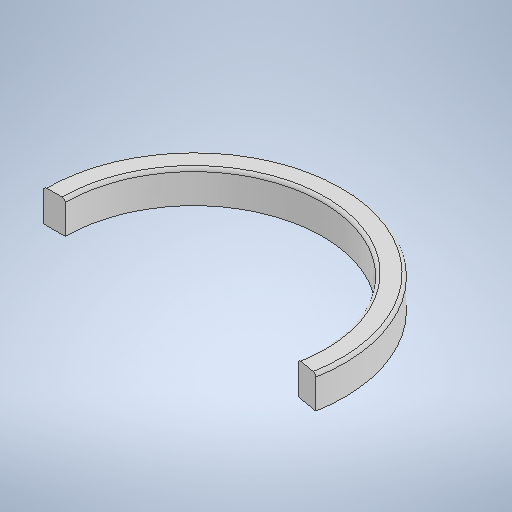
# Autodesk Inventor part: InertiaKitInner
Saved by Autodesk Inventor 2025 (Build 290162000, 162)
## iProperties
Created: 2026-01-08
Part Number: InertiaKitInner
Material: Generic
Document SubType Name: Modeling
Designer: tapen
Density: 1 g/cm^3
Appearance: Default
Author: tapen
Autodesk Inventor part; units mm, degrees
ref_plane "YZ Plane" through (0, 0, 0) normal (1, 0, 0) x (0, 1, 0)
ref_plane "XZ Plane" through (0, 0, 0) normal (0, 1, 0) x (-1, 0, 0)
ref_plane "XY Plane" through (0, 0, 0) normal (0, 0, 1) x (1, 0, 0)
sketch "Sketch1" plane through (0, 0, 0) normal (0, 0, 1) x (1, 0, 0)
  line L0 (7, 0) -> (7, 19)
  line L1 (7, 0) -> (26, 0) construction
  line L2 (5, 21) -> (-5, 21)
  line L3 (-7, 19) -> (-7, 0)
  line L4 (-7, 0) -> (7, 0)
  arc A0 (-5, 21) -> (-7, 19) centre (-5, 19) ccw
  arc A1 (7, 19) -> (5, 21) centre (5, 19) ccw
  line L5 (90, 15.1029) -> (90, 0) construction
  point P0 (0, 0)
  point P1 (7, 21)
  point P2 (-7, 21)
  point P3 (0, 0)
  dimension "d0" = 21
  dimension "d1" = 90
  dimension "d2" = 7
  dimension "d3" = 14
  dimension "d4" = 2
  dimension "d5" = 90
  constraints: 12 end point, 4 point on circle, 4 point on line, 4 tangent, 2 centre point, 2 horizontal, 2 perpendicular, 2 vertical, 1 collinear, 1 equal radius, 1 midpoint
  measures "d0" distance of L0.start point (7, 21)
  measures "d1" angle of L1 L0
  measures "d2" distance from line of L0 point (0, 0)
  measures "d3" distance of point (7, 21) point (-7, 21)
  measures "d4" radius of A0
  measures "d5" distance from line of point (0, 0) L5
revolve "Revolution1" add sketch "Sketch1" angle 190 about axis through (90, 15.1029, 0) along (0, -1, 0)
body "Solid1"
